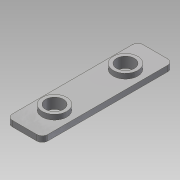
# Autodesk Inventor part: Double T-Nut
Saved by Autodesk Inventor 2013 SP2 (Build 170200200, 200)
## iProperties
Created: 2013-07-08
Part Number: Double T-Nut
Material: Steel
Document SubType Name: Modeling
Designer: Jon Hollander
Density: 7.85 g/cm^3
Mass: 4.50463 g
Surface Area: 9.55957 cm^2
Volume: 0.573839 cm^3
Author: Jon Hollander
Autodesk Inventor part; units mm, degrees
ref_plane "YZ Plane" through (0, 0, 0) normal (1, 0, 0) x (0, 1, 0)
ref_plane "XZ Plane" through (0, 0, 0) normal (0, 1, 0) x (-1, 0, 0)
ref_plane "XY Plane" through (0, 0, 0) normal (0, 0, 1) x (1, 0, 0)
sketch "Sketch1" plane through (0, 0, 0) normal (0, 0, 1) x (1, 0, 0)
  line L0 (-5, -18.44) -> (5, -18.44)
  line L1 (5, -18.44) -> (5, 18.44)
  line L2 (5, 18.44) -> (-5, 18.44)
  line L3 (-5, 18.44) -> (-5, -18.44)
  line L4 (-5, -18.44) -> (5, 18.44) construction
  line L5 (5, -18.44) -> (-5, 18.44) construction
  point P0 (0, 0)
  dimension "d0" = 10
  dimension "d1" = 36.88
  constraints: 12 end point, 2 midpoint, 2 parallel, 1 horizontal, 1 perpendicular
  measures "d0" distance of L2.end L1.end
  measures "d1" distance of L0.end L1.end
extrude "Extrusion1" add sketch "Sketch1" along normal blind 1.6
sketch "Sketch2" plane through (0, 0, 1.6) normal (0, 0, 1) x (1, 0, 0)
  line L0 (5, -18.44) -> (5, 18.44) projected
  line L1 (5, 18.44) -> (-5, 18.44) projected
  line L2 (-5, 18.44) -> (-5, -18.44) projected
  line L3 (-5, 0) -> (5, 0) construction
  circle A0 centre (0, 10) radius 3.45
  circle A1 centre (0, -10) radius 3.45
  point P0 (0, 0)
  dimension "d5" = 6.9
  dimension "d7" = 8.44
  dimension "d8" = 5
  constraints: 2 centre point, 2 end point, 2 midpoint, 1 symmetric about line, 1 other
  measures "d5" diameter of A0
  measures "d7" distance from line of L1 A0.centre
  measures "d8" distance from line of A0.centre L0
extrude "Extrusion2" add sketch "Sketch2" along normal blind 1.4
sketch "Sketch3" plane through (0, -10, 3) normal (0, 0, 1) x (1, 0, 0)
  circle A0 centre (0, 0) radius 3.45 projected
  circle A1 centre (0, 20) radius 3.45 projected
  point P0 (0, 10)
  constraints: 2 coincident
hole "Hole1" at (0, -10, 3) at (0, 10, 3) direction (0, 0, -1) diameter 5 end through all
fillet "Fillet1" radius 1.51 4 edges at (5, 18.44, 0.8) (-5, 18.44, 0.8) (-5, -18.44, 0.8) (5, -18.44, 0.8)
body "Solid1"
